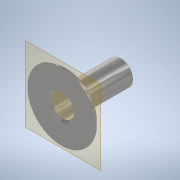
# Autodesk Inventor part: dekiel
Saved by Autodesk Inventor 2021 (Build 250183000, 183)
## iProperties
Created: 2021-05-20
Part Number: dekiel
Material: Stal nierdzewna
Document SubType Name: Modeling
Designer: Wojciech Wołczek
Density: 8 g/cm^3
Appearance: Częściowo polerowana
Mass: 1832.7 g
Surface Area: 1217.78 cm^2
Volume: 229.088 cm^3
Author: Wojciech Wołczek
Autodesk Inventor part; units mm, degrees
ref_plane "YZ Plane" through (0, 0, 0) normal (1, 0, 0) x (0, 1, 0)
ref_plane "XZ Plane" through (0, 0, 0) normal (0, 1, 0) x (-1, 0, 0)
ref_plane "XY Plane" through (0, 0, 0) normal (0, 0, 1) x (1, 0, 0)
ref_plane "Płaszczyzna konstrukcyjna1" through (0, 0, 0) normal (0, 0, 1) x (1, 0, 0)
sketch "Szkic1" plane through (0, 0, 0) normal (0, 0, 1) x (1, 0, 0)
  circle A0 centre (90, 0) radius 90 projected
  circle A1 centre (90, 0) radius 80 projected
  circle A2 centre (90, 0) radius 80
  circle A3 centre (90, 0) radius 72.5
  circle A4 centre (90, 0) radius 30
  point P0 (0, 0)
  dimension "d0" = 145
  dimension "d1" = 60
  constraints: 3 centre point, 3 coincident, 1 concentric, 1 horizontal alignment
  measures "d0" diameter of A3
  measures "d1" diameter of A4
extrude "Wyciągnięcie proste1" add sketch "Szkic1" along normal blind 5 contours A0 | A1 | A3
sketch "Szkic2" plane through (90, 0, 0) normal (0, 0, -1) x (-1, 0, 0)
  circle A0 centre (0, 0) radius 30
  circle A1 centre (0, 0) radius 32.5
  point P0 (90, 0)
  dimension "d4" = 65
  constraints: 2 centre point, 1 coincident
  measures "d4" diameter of A1
extrude "Wyciągnięcie proste2" add sketch "Szkic2" along normal blind 150
sketch "Szkic3" plane through (90, 0, -150) normal (0, 0, -1) x (-1, 0, 0)
  circle A0 centre (0, 0) radius 32.5
  point P0 (90, 0)
  constraints: 1 centre point
extrude "Wyciągnięcie proste3" add sketch "Szkic3" along normal blind 3
chamfer "Faza1" distance 1 angle 45 1 edges at (122.5, 0, -153)
chamfer "Faza2" distance 5 angle 45 1 edges at (60, 0, 5)
sketch "Szkic4" plane through (90, 0, 0) normal (0, 0, -1) x (-1, 0, 0)
  circle A0 centre (0, 0) radius 80 projected
  circle A1 centre (0, 0) radius 80
  circle A2 centre (0, 0) radius 72.5
  point P0 (90, 0)
  dimension "d15" = 145
  constraints: 2 centre point, 2 coincident, 1 concentric
  measures "d15" diameter of A2
extrude "Wyciągnięcie proste4" add sketch "Szkic4" along normal blind 10
chamfer "Faza3" distance 1 angle 45 5 edges at (0, 0, 5) (0, 0, 0) (170, 0, -10) (162.5, 0, -10) (122.5, 0, 0)
